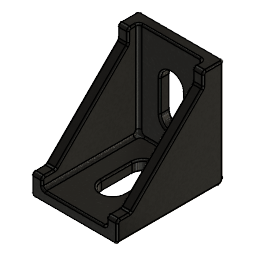
_3030 Angle Bracket.8fdec9af-f8a9-4786-83be-04986f9cd556 (Autodesk Fusion 360 design; units mm, degrees)
Autodesk Fusion 360 part; units mm, degrees
sketch "Sketch1" plane through (0, 0, 0) normal (0, 1, 0) x (1, 0, 0)
  line L0 (0, 0) -> (28, 0)
  line L1 (28, 0) -> (28, -35)
  line L2 (28, -35) -> (0, -35)
  line L3 (0, -35) -> (0, 0)
  line L4 (0, -3.5) -> (28, -3.5) construction
  line L5 (10.35, -12.5) -> (10.35, -22.5)
  arc A0 (10.35, -22.5) -> (17.65, -22.5) centre (14, -22.5) ccw
  line L6 (17.65, -22.5) -> (17.65, -12.5)
  arc A1 (17.65, -12.5) -> (10.35, -12.5) centre (14, -12.5) ccw
  line L7 (14, -12.5) -> (14, -22.5) construction
  point P0 (14, -35)
  point P1 (14, -17.5)
  point P2 (28, -17.5)
  dimension "d1" = 28
  dimension "d2" = 35
  dimension "d3" = 3.5
  dimension "d4" = 3.65
  dimension "d5" = 10
  constraint horizontal L0
  constraint vertical L1
  constraint horizontal L2
  constraint vertical L3
  constraint coincident L0.start L3.end
  constraint coincident L3 L4.start
  constraint coincident L1 L4.end
  constraint perpendicular L1 L4
  constraint tangent L5 A0
  constraint tangent A0 L6
  constraint parallel L5 L6
  constraint tangent L6 A1
  constraint tangent L5 A1
  constraint perpendicular L2 L7
  constraint midpoint L2 P0
  constraint vertical A0.centre P0
  constraint midpoint L7 P1
  constraint midpoint L1 P2
  constraint horizontal P1 P2
  measures "d1" distance of L0.start L0.end
  measures "d2" distance of L0.start L2.end
  measures "d3" distance of L0 L4
  measures "d4" radius of A0
  measures "d5" distance of A1.centre A0.centre
extrude "Extrude1" add sketch "Sketch1" along normal blind 3.5
sketch "Sketch2" plane through (0, 0, 0) normal (0, 0, -1) x (1, 0, 0)
  line L0 (28, 0) -> (0, 0)
  line L1 (0, 0) -> (0, -3.5)
  line L2 (0, -3.5) -> (28, -3.5)
  line L3 (28, -3.5) -> (28, 0)
  line L4 (0, -3.5) -> (28, -3.5)
  line L5 (28, -3.5) -> (28, 31.5)
  line L6 (28, 31.5) -> (0, 31.5)
  line L7 (0, 31.5) -> (0, -3.5)
  line L8 (17.65, 9) -> (17.65, 19)
  arc A0 (17.65, 19) -> (10.35, 19) centre (14, 19) ccw
  line L9 (10.35, 19) -> (10.35, 9)
  arc A1 (10.35, 9) -> (17.65, 9) centre (14, 9) ccw
  line L10 (14, 9) -> (14, 19) construction
  point P0 (28, -3.5)
  point P1 (0, -3.5)
  point P2 (14, 31.5)
  point P3 (14, 14)
  point P4 (28, 14)
  dimension "d8" = 28
  dimension "d9" = 35
  dimension "d10" = 7.3
  dimension "d11" = 10
  constraint horizontal L4
  constraint vertical L5
  constraint horizontal L6
  constraint vertical L7
  constraint coincident P1 L1.end
  constraint tangent L8 A0
  constraint tangent A0 L9
  constraint parallel L8 L9
  constraint tangent L9 A1
  constraint tangent L8 A1
  constraint perpendicular L6 L10
  constraint midpoint L6 P2
  constraint vertical A0.centre P2
  constraint midpoint L10 P3
  constraint midpoint L5 P4
  constraint horizontal P3 P4
  measures "d8" distance of P1 P0
  measures "d9" distance of P1 L6.end
  measures "d10" diameter of A0
  measures "d11" distance of A1.centre A0.centre
extrude "Extrude2" add sketch "Sketch2" against normal blind 3.5 contours L0 L5 L6 L7
sketch "Sketch3" plane through (0, 0, 0) normal (-1, 0, 0) x (0, -1, 0)
  line L0 (0, 3.5) -> (0, 35)
  line L1 (0, 35) -> (-3.5, 35)
  line L2 (-3.5, 35) -> (-3.5, 0)
  line L3 (-3.5, 0) -> (31.5, 0)
  line L4 (31.5, 0) -> (31.5, 3.5)
  line L5 (31.5, 3.5) -> (0, 3.5)
  line L6 (0, 35) -> (3.5, 35)
  line L7 (3.5, 35) -> (3.5, 30.5)
  line L8 (3.5, 30.5) -> (27, 7)
  line L9 (27, 7) -> (31.5, 7)
  line L10 (31.5, 7) -> (31.5, 3.5)
  line L11 (0, 3.5) -> (15.25, 18.75) construction
  dimension "d14" = 45
  dimension "d15" = 3.5
  dimension "d16" = 4.5
  constraint coincident L0.end L1.start
  constraint perpendicular L0 L6
  constraint perpendicular L6 L7
  constraint parallel L6 L9
  constraint coincident L4.end L5.start
  constraint vertical L10
  constraint coincident L0.start L5.end
  constraint midpoint L8 L11.end
  constraint symmetric L7 L9 L11
  measures "d14" angle of L5 L11
  measures "d15" distance of L9.end L4.end
  measures "d16" distance of L8.end L9.end
extrude "Extrude3" add sketch "Sketch3" against normal blind 3.5 contours L0 L5 L6 L7 L8 L9 L10
sketch "Sketch4" plane through (28, 0, 0) normal (1, 0, 0) x (0, 1, 0)
  line L0 (-31.5, 0) -> (3.5, 0)
  line L1 (3.5, 0) -> (3.5, 35)
  line L2 (3.5, 35) -> (0, 35)
  line L3 (0, 35) -> (0, 3.5)
  line L4 (0, 3.5) -> (-31.5, 3.5)
  line L5 (-31.5, 3.5) -> (-31.5, 0)
  line L6 (-27, 7) -> (-31.5, 7)
  line L7 (-31.5, 7) -> (-31.5, 3.5)
  line L8 (-31.5, 3.5) -> (0, 3.5)
  line L9 (0, 3.5) -> (0, 35)
  line L10 (0, 35) -> (-3.5, 35)
  line L11 (-3.5, 35) -> (-3.5, 30.5)
  line L12 (-3.5, 30.5) -> (-27, 7)
extrude "Extrude4" add sketch "Sketch4" against normal blind 3.5 contours L3 L4 L6 L7 L8 L9 L10 L11 L12
fillet "Fillet1" radius 1 4 edges at (1.75, -31.5, 7) (1.75, -3.5, 35) (26.25, -3.5, 35) (26.25, -31.5, 7)
fillet "Fillet1" radius 1 4 edges at (26.25, -3.5, 30.5) (26.25, -27, 7) (1.75, -27, 7) (1.75, -3.5, 30.5)
fillet "Fillet1" radius 1 8 edges at (28, 3.5, 17.5) (24.5, 0, 19.25) (3.5, 0, 19.25) (0, 3.5, 17.5) (24.5, -15.75, 3.5) (28, -14, 0) (3.5, -15.75, 3.5) (0, -14, 0)
fillet "Fillet1" radius 0.5 42 edges at (14, -31.5, 0) (14, -31.5, 3.5) (14, 0, 35) (14, 3.5, 35) (24.5, -1.75, 35) (3.5, -1.75, 35) (3.5, -29.25, 7) (24.5, -29.25, 7) (24.5, -31.5, 5.25) (3.5, -31.5, 5.25) (24.5, -3.5, 32.75) (3.5, -3.5, 32.75) (0, -15.25, 18.75) (3.5, -15.25, 18.75) (24.5, -15.25, 18.75) (28, -15.25, 18.75) (28, -31.5, 3.5) (28, -29.25, 7) (0, -29.25, 7) (0, -31.5, 3.5) (0, 0, 35) (28, 0, 35) (28, -3.5, 32.75) (0, -3.5, 32.75) (14, 3.5, 0) (14, 0, 3.5) (14, 0, 26.15) (10.35, 0, 17.5) (14, 0, 8.85) (17.65, 0, 17.5) (14, 3.5, 26.15) (10.35, 3.5, 17.5) (14, 3.5, 8.85) (17.65, 3.5, 17.5) (14, -22.65, 3.5) (10.35, -14, 3.5) (14, -5.35, 3.5) (17.65, -14, 3.5) (14, -22.65, 0) (17.65, -14, 0) (14, -5.35, 0) (10.35, -14, 0)
equation "d4 = ( 7.3 / 2 ) * 1 mm"
